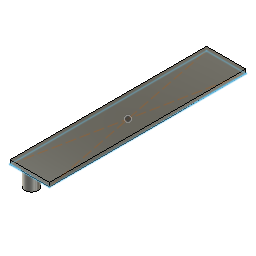
futa (Autodesk Fusion 360 design; units mm, degrees)
Autodesk Fusion 360 part; units mm, degrees
sketch "スケッチ1" plane through (0, 0, 0) normal (0, 0, 1) x (1, 0, 0)
  line L0 (15, -75) -> (-15, 75) construction
  line L1 (-15, -75) -> (-15, 75)
  line L2 (-15, -75) -> (15, 75) construction
  line L3 (15, 75) -> (15, -75)
  line L4 (-15, 75) -> (15, 75)
  line L5 (15, -75) -> (-15, -75)
  dimension "d1" = 150
  dimension "d2" = 30
  constraint horizontal L5
  constraint perpendicular L1 L5
  constraint parallel L4 L5
  constraint parallel L1 L3
  constraint coincident origin L0
  constraint coincident origin L2
  measures "d1" distance of L0.end L1.start
  measures "d2" distance of L2.end L0.end
extrude "押し出し1" add sketch "スケッチ1" along normal blind 3 makes body 1
sketch "スケッチ2" plane through (0, 0, 0) normal (0, 0, 1) x (1, 0, 0)
  circle A0 centre (-7.0403, -66.7625) radius 5
  dimension "d5" = 10
  measures "d5" diameter of A0
extrude "押し出し2" add sketch "スケッチ2" against normal blind 15 separate body makes body 2
